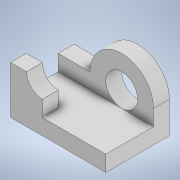
# Autodesk Inventor part: 零件7
Saved by Autodesk Inventor 2020 (Build 240168000, 168)
## iProperties
Created: 2020-09-19
Part Number: 零件7
Material: 一般
Document SubType Name: Modeling
Designer: User
Density: 1 g/cm^3
Appearance: 預設
Author: User
Autodesk Inventor part; units mm, degrees
ref_plane "YZ Plane" through (0, 0, 0) normal (1, 0, 0) x (0, 1, 0)
ref_plane "XZ Plane" through (0, 0, 0) normal (0, 1, 0) x (-1, 0, 0)
ref_plane "XY Plane" through (0, 0, 0) normal (0, 0, 1) x (1, 0, 0)
sketch "草圖1" plane through (0, 0, 0) normal (0, 0, 1) x (1, 0, 0)
  line L0 (0, 0) -> (60, 0)
  line L1 (60, 0) -> (60, 10)
  line L2 (60, 10) -> (0, 10)
  line L3 (0, 10) -> (0, 0)
  circle A0 centre (40, 20) radius 10
  arc A1 (60, 20) -> (20, 20) centre (40, 20) ccw
  line L4 (20, 20) -> (20, 10)
  line L5 (60, 20) -> (60, 10)
  line L6 (20, 10) -> (0, 10)
  line L7 (0, 10) -> (0, 20)
  line L8 (0, 20) -> (20, 20)
  line L9 (20, 20) -> (20, 10)
  point P0 (40, 10)
  dimension "d0" = 60
  dimension "d1" = 10
  dimension "d2" = 20
  dimension "d3" = 40
  dimension "d4" = 10
  dimension "d5" = 20
  dimension "d10" = 20
  dimension "d11" = 10
  constraints: 20 end point, 4 parallel, 3 perpendicular, 2 centre point, 2 horizontal, 2 point on circle, 1 coincident, 1 point on line, 1 tangent
  measures "d0" distance of L2.end L1.end
  measures "d1" distance of L1.end L0.end
  measures "d2" diameter of A0
  measures "d3" diameter of A1
  measures "d4" distance from line of L2 A0.centre
  measures "d5" distance from line of L1 A0.centre
  measures "d10" distance of L7.end L8.end
  measures "d11" distance of L6.end L7.end
extrude "擠出1" add sketch "草圖1" along normal blind 10 contours L7 L8 L4 L2 | L2 L4 A1 L5
extrude "擠出2" add sketch "草圖1" along normal blind 40 contours L3 L2 L1 L0
sketch "草圖2" plane through (0, 0, 40) normal (0, 0, 1) x (1, 0, 0)
  line L0 (0, 10) -> (0, 0) projected
  line L1 (0, 10) -> (20, 10)
  line L2 (20, 10) -> (20, 20)
  line L3 (10, 30) -> (0, 30)
  line L4 (0, 30) -> (0, 10)
  arc A0 (10, 30) -> (20, 20) centre (20, 30) ccw
  constraints: 8 end point, 2 parallel, 2 point on circle, 1 centre point, 1 horizontal, 1 perpendicular
extrude "擠出3" add sketch "草圖2" against normal blind 10
